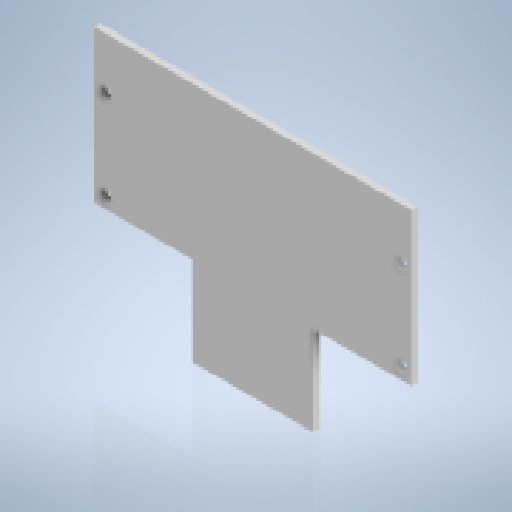
# Autodesk Inventor part: pokrywa
Saved by Autodesk Inventor 2023 (Build 270158000, 158)
## iProperties
Created: 2025-01-11
Part Number: pokrywa
Material: Ogólny
Document SubType Name: Modeling
Designer: kamil
Density: 1 g/cm^3
Appearance: Domyślna
Author: kamil
Autodesk Inventor part; units mm, degrees
ref_plane "YZ Plane" through (0, 0, 0) normal (1, 0, 0) x (0, 1, 0)
ref_plane "XZ Plane" through (0, 0, 0) normal (0, 1, 0) x (-1, 0, 0)
ref_plane "XY Plane" through (0, 0, 0) normal (0, 0, 1) x (1, 0, 0)
sketch "Szkic1" plane through (0, 0, 0) normal (0, 0, 1) x (1, 0, 0)
  line L0 (54, -15.2042) -> (54, -5) projected
  line L1 (18, -31) -> (52, -31) projected
  circle A0 centre (35, -25.5) radius 3.5 projected
  circle A1 centre (26, -7) radius 3.5 projected
  circle A2 centre (44, -7) radius 3.5 projected
  line L2 (18, -31) -> (52, -31) projected
  line L3 (54, -24.7958) -> (54, -29) projected
  line L4 (54, -15.2042) -> (54, -5) projected
  line L5 (52, -3) -> (18, -3) projected
  line L6 (16, -5) -> (16, -15.2042) projected
  line L7 (16, -24.7958) -> (16, -20) projected
  line L8 (85, -3) -> (85, 41.8489) projected
  line L9 (-15, 44.8489) -> (85, 44.8489) projected
  line L10 (-15, -3) -> (-15, 41.8489) projected
  line L11 (-15, -4) -> (15.8, -4)
  line L12 (85, 44.8489) -> (-15, 44.8489)
  line L13 (-15, 44.8489) -> (-15, -3)
  line L14 (-15, -3) -> (85, -3)
  line L15 (85, -3) -> (85, 44.8489)
  line L16 (52, -31) -> (16, -31)
  line L17 (16, -31) -> (16, -3)
  line L18 (16, -3) -> (52, -3)
  line L19 (52, -3) -> (52, -31)
  arc A3 (54, -5) -> (52, -3) centre (52, -5) ccw projected
  arc A4 (18, -3) -> (16, -5) centre (18, -5) ccw projected
  line L20 (16, -15.2042) -> (16, -20) projected
  line L21 (16, -29) -> (16, -24.7958) projected
  arc A5 (16, -29) -> (18, -31) centre (18, -29) ccw projected
  arc A6 (52, -31) -> (54, -29) centre (52, -29) ccw projected
  line L22 (54, -15.2042) -> (54, -24.7958) projected
  line L23 (54, -15.2042) -> (54, -15.2042) projected
  point P0 (0, 0)
  point P1 (54, -3)
  point P2 (52, -3)
  constraints: 18 end point, 4 parallel, 3 horizontal, 2 perpendicular, 2 other
extrude "Wyciągnięcie proste1" add sketch "Szkic1" along normal blind 2 contours L5 L14 L10 L13 L9 L15 L8
sketch "Szkic2" plane through (0, 0, 2) normal (0, 0, 1) x (1, 0, 0)
  circle A0 centre (81.5, 0.5) radius 2 projected
  circle A1 centre (81.5, 28.3844) radius 2 projected
  circle A2 centre (-11.5, 28.3844) radius 2 projected
  circle A3 centre (-11.5, 0.5) radius 2 projected
  point P0 (0, 0)
hole "Otwór1" at (81.5, 0.5, 2) at (81.5, 28.3844, 2) at (-11.5, 0.5, 2) at (-11.5, 28.3844, 2) direction (0, 0, -1) diameter 3.2 depth 7 tip angle 118 countersink diameter 3.8 countersink angle 90
sketch "Szkic3" plane through (0, 0, 2) normal (0, 0, 1) x (1, 0, 0)
  circle A0 centre (35, -25.5) radius 3.5 projected
  circle A1 centre (26, -7) radius 3.5 projected
  circle A2 centre (44, -7) radius 3.5 projected
  arc A3 (54, -5) -> (52, -3) centre (52, -5) ccw projected
  line L0 (52, -3) -> (18, -3) projected
  arc A4 (18, -3) -> (16, -5) centre (18, -5) ccw projected
  line L1 (16, -5) -> (16, -15.2042) projected
  line L2 (16, -15.2042) -> (16, -20) projected
  line L3 (16, -24.7958) -> (16, -20) projected
  line L4 (16, -29) -> (16, -24.7958) projected
  arc A5 (16, -29) -> (18, -31) centre (18, -29) ccw projected
  line L5 (18, -31) -> (52, -31) projected
  arc A6 (52, -31) -> (54, -29) centre (52, -29) ccw projected
  line L6 (54, -24.7958) -> (54, -29) projected
  line L7 (54, -20) -> (54, -24.7958) projected
  line L8 (54, -20) -> (54, -15.2042) projected
  line L9 (54, -15.2042) -> (54, -5) projected
  circle A7 centre (-11.5, 0.5) radius 1.9 projected
  circle A8 centre (81.5, 0.5) radius 1.9 projected
  circle A9 centre (81.5, 28.3844) radius 1.9 projected
  circle A10 centre (-11.5, 28.3844) radius 1.9 projected
  line L10 (85, 44.8489) -> (-15, 44.8489) projected
  line L11 (-15, 44.8489) -> (-15, -3) projected
  line L12 (-15, -3) -> (85, -3) projected
  line L13 (85, -3) -> (85, 44.8489) projected
  line L14 (16, -5) -> (16, -3)
  line L15 (54, -5) -> (54, -3)
  point P0 (0, 0)
  point P1 (52, -3)
  constraints: 4 end point, 2 perpendicular, 2 point on line
extrude "Wyciągnięcie proste2" add sketch "Szkic3" against normal up to surface (2 mm away) contours A0 | A1 | A2 | L9 L8 L7 L6 A6 L5 A5 L4 L3 L2 L1 A4 L0 A3 | A3 L12 L15 | A4 L14 L12
fillet "Zaokrąglenie1" radius 2 6 edges at (85, -3, 1) (54, -3, 1) (85, 44.8489, 1) (16, -3, 1) (-15, -3, 1) (-15, 44.8489, 1)
